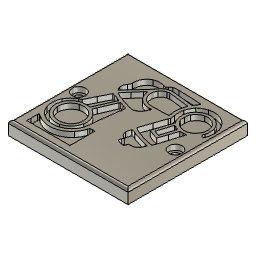
logo negative (Autodesk Fusion 360 design; units mm, degrees)
Autodesk Fusion 360 part; units mm, degrees
(part 1 of 2)
sketch "Sketch1" plane through (0, 0, 0) normal (0, 0, 1) x (1, 0, 0)
  line L0 (0, 0) -> (45, 0)
  line L1 (45, 0) -> (45, 45)
  line L2 (45, 45) -> (0, 45)
  line L3 (0, 45) -> (0, 0)
  dimension "d1" = 45
  dimension "d2" = 45
  constraint horizontal L0
  constraint vertical L1
  constraint horizontal L2
  constraint vertical L3
  constraint coincident L0.start L3.end
  measures "d1" distance of L0.start L0.end
  measures "d2" distance of L0.start L2.end
extrude "Extrude1" add sketch "Sketch1" along normal blind 5
sketch "Sketch2" plane through (0, 0, 5) normal (0, 0, 1) x (-1, 0, 0)
  line L0 (0, -45) -> (0, 0)
  line L1 (0, 0) -> (-45, 0)
  line L2 (-45, 0) -> (-45, -45)
  line L3 (-45, -45) -> (0, -45)
  spline S0 degree 3 poles (-20.168, -41.6441) (-19.9884, -41.5159) (-19.6164, -41.208) (-19.3214, -40.9258) knots 0 0 0 0 1 1 1 1
  line L4 (-19.3214, -40.9258) -> (-18.7954, -40.4255)
  line L5 (-18.7954, -40.4255) -> (-17.782, -40.6436)
  spline S1 degree 3 poles (-17.782, -40.6436) (-16.371, -40.9386) (-14.9471, -40.8488) (-13.985, -40.4127) knots 0 0 0 0 1 1 1 1
  spline S2 degree 3 poles (-13.985, -40.4127) (-12.2276, -39.6045) (-11.2014, -37.8086) (-11.1886, -35.5124) knots 0 0 0 0 1 1 1 1
  spline S3 degree 3 poles (-11.1886, -35.5124) (-11.1757, -34.9737) (-11.0988, -34.7299) (-10.6754, -34.1014) knots 0 0 0 0 1 1 1 1
  spline S4 degree 3 poles (-10.6754, -34.1014) (-10.1495, -33.3061) (-9.9443, -32.5236) (-10.0854, -31.8309) knots 0 0 0 0 1 1 1 1
  spline S5 degree 3 poles (-10.0854, -31.8309) (-10.1752, -31.3306) (-10.5472, -30.5609) (-10.6754, -30.5609) knots 0 0 0 0 1 1 1 1
  spline S6 degree 3 poles (-10.6754, -30.5609) (-10.7396, -30.5609) (-11.4964, -31.3178) (-12.3687, -32.2542) knots 0 0 0 0 1 1 1 1
  spline S7 degree 3 poles (-12.3687, -32.2542) (-13.241, -33.1778) (-14.5751, -34.6017) (-15.3319, -35.4098) knots 0 0 0 0 1 1 1 1
  spline S8 degree 3 poles (-15.3319, -35.4098) (-16.1016, -36.218) (-17.038, -37.2955) (-17.41, -37.8086) knots 0 0 0 0 1 1 1 1
  spline S9 degree 3 poles (-17.41, -37.8086) (-18.1797, -38.8477) (-19.052, -39.6558) (-19.7575, -40.0022) knots 0 0 0 0 1 1 1 1
  spline S10 degree 3 poles (-19.7575, -40.0022) (-20.5272, -40.3742) (-21.6689, -40.3614) (-25.1709, -39.938) knots 0 0 0 0 1 1 1 1
  spline S11 degree 3 poles (-25.1709, -39.938) (-26.9668, -39.72) (-28.737, -39.5019) (-29.0833, -39.4634) knots 0 0 0 0 1 1 1 1
  line L6 (-29.0833, -39.4634) -> (-29.7247, -39.3993)
  line L7 (-29.7247, -39.3993) -> (-30.3918, -40.3998)
  spline S12 degree 3 poles (-30.3918, -40.3998) (-30.969, -41.2593) (-31.0332, -41.4132) (-30.8408, -41.4774) knots 0 0 0 0 1 1 1 1
  spline S13 degree 3 poles (-30.8408, -41.4774) (-30.5329, -41.5928) (-24.7091, -41.8494) (-22.4001, -41.8494) knots 0 0 0 0 1 1 1 1
  spline S14 degree 3 poles (-22.4001, -41.8494) (-20.8351, -41.8494) (-20.4246, -41.8109) (-20.168, -41.6441) knots 0 0 0 0 1 1 1 1
  spline S15 degree 3 poles (-34.2786, -41.0412) (-33.1113, -40.6949) (-31.8798, -39.9637) (-31.2769, -39.271) knots 0 0 0 0 1 1 1 1
  spline S16 degree 3 poles (-31.2769, -39.271) (-30.6868, -38.5655) (-29.9685, -37.1801) (-29.7247, -36.2565) knots 0 0 0 0 1 1 1 1
  spline S17 degree 3 poles (-29.7247, -36.2565) (-29.5067, -35.4227) (-29.481, -33.7422) (-29.6734, -32.8699) knots 0 0 0 0 1 1 1 1
  spline S18 degree 3 poles (-29.6734, -32.8699) (-29.9172, -31.7539) (-29.9428, -31.3306) (-29.8145, -31.1766) knots 0 0 0 0 1 1 1 1
  spline S19 degree 3 poles (-29.8145, -31.1766) (-29.7504, -31.0869) (-29.6221, -30.8046) (-29.558, -30.5609) knots 0 0 0 0 1 1 1 1
  spline S20 degree 3 poles (-29.558, -30.5609) (-29.481, -30.3172) (-28.8396, -28.4058) (-28.1213, -26.3277) knots 0 0 0 0 1 1 1 1
  spline S21 degree 3 poles (-28.1213, -26.3277) (-26.7359, -22.3126) (-26.5434, -21.6969) (-26.6076, -21.6584) knots 0 0 0 0 1 1 1 1
  spline S22 degree 3 poles (-26.6076, -21.6584) (-27.3131, -21.1453) (-29.6991, -20.1576) (-31.4693, -19.6444) knots 0 0 0 0 1 1 1 1
  spline S23 degree 3 poles (-31.4693, -19.6444) (-32.9958, -19.2083) (-34.8559, -18.8363) (-35.0739, -18.9261) knots 0 0 0 0 1 1 1 1
  spline S24 degree 3 poles (-35.0739, -18.9261) (-35.2407, -18.9902) (-35.4973, -19.6829) (-36.3311, -22.4794) knots 0 0 0 0 1 1 1 1
  spline S25 degree 3 poles (-36.3311, -22.4794) (-36.5491, -23.2234) (-36.78, -23.9674) (-36.8442, -24.147) knots 0 0 0 0 1 1 1 1
  spline S26 degree 3 poles (-36.8442, -24.147) (-36.9083, -24.3266) (-37.1007, -24.9936) (-37.2931, -25.6222) knots 0 0 0 0 1 1 1 1
  spline S27 degree 3 poles (-37.2931, -25.6222) (-37.4856, -26.2636) (-37.7806, -27.2257) (-37.9602, -27.7901) knots 0 0 0 0 1 1 1 1
  spline S28 degree 3 poles (-37.9602, -27.7901) (-38.127, -28.3417) (-38.2424, -28.8163) (-38.2167, -28.8548) knots 0 0 0 0 1 1 1 1
  spline S29 degree 3 poles (-38.2167, -28.8548) (-38.1783, -28.8805) (-37.6395, -28.842) (-36.9981, -28.7522) knots 0 0 0 0 1 1 1 1
  line L8 (-36.9981, -28.7522) -> (-35.8436, -28.6111)
  line L9 (-35.8436, -28.6111) -> (-34.8045, -25.417)
  spline S30 degree 3 poles (-34.8045, -25.417) (-34.2273, -23.6724) (-33.7142, -22.21) (-33.6629, -22.1715) knots 0 0 0 0 1 1 1 1
  spline S31 degree 3 poles (-33.6629, -22.1715) (-33.5346, -22.0946) (-30.1865, -23.1849) (-30.0198, -23.3517) knots 0 0 0 0 1 1 1 1
  spline S32 degree 3 poles (-30.0198, -23.3517) (-29.93, -23.4415) (-30.3148, -24.7756) (-31.0588, -27.0076) knots 0 0 0 0 1 1 1 1
  line L10 (-31.0588, -27.0076) -> (-32.2262, -30.5353)
  line L11 (-32.2262, -30.5353) -> (-31.9055, -31.0869)
  spline S33 degree 3 poles (-31.9055, -31.0869) (-31.123, -32.4594) (-30.8536, -34.3964) (-31.2641, -35.769) knots 0 0 0 0 1 1 1 1
  spline S34 degree 3 poles (-31.2641, -35.769) (-31.713, -37.2827) (-33.3037, -38.7964) (-34.9457, -39.2966) knots 0 0 0 0 1 1 1 1
  spline S35 degree 3 poles (-34.9457, -39.2966) (-35.9077, -39.5917) (-37.306, -39.5917) (-38.2809, -39.2966) knots 0 0 0 0 1 1 1 1
  spline S36 degree 3 poles (-38.2809, -39.2966) (-39.5637, -38.899) (-40.9362, -37.5649) (-41.5007, -36.1667) knots 0 0 0 0 1 1 1 1
  spline S37 degree 3 poles (-41.5007, -36.1667) (-41.847, -35.32) (-41.8727, -33.3574) (-41.5391, -32.4979) knots 0 0 0 0 1 1 1 1
  spline S38 degree 3 poles (-41.5391, -32.4979) (-41.2185, -31.6384) (-41.2698, -31.4075) (-41.7829, -31.1638) knots 0 0 0 0 1 1 1 1
  spline S39 degree 3 poles (-41.7829, -31.1638) (-42.0394, -31.0484) (-42.2575, -30.9457) (-42.2832, -30.9457) knots 0 0 0 0 1 1 1 1
  spline S40 degree 3 poles (-42.2832, -30.9457) (-42.3088, -30.9457) (-42.5012, -31.3306) (-42.6937, -31.818) knots 0 0 0 0 1 1 1 1
  spline S41 degree 3 poles (-42.6937, -31.818) (-43.04, -32.6134) (-43.0657, -32.793) (-43.0528, -34.281) knots 0 0 0 0 1 1 1 1
  spline S42 degree 3 poles (-43.0528, -34.281) (-43.04, -35.6536) (-42.9887, -36.0127) (-42.7321, -36.7183) knots 0 0 0 0 1 1 1 1
  spline S43 degree 3 poles (-42.7321, -36.7183) (-41.4237, -40.2074) (-37.7806, -42.0675) (-34.2786, -41.0412) knots 0 0 0 0 1 1 1 1
  spline S44 degree 3 poles (-20.5657, -39.1299) (-19.8986, -38.9503) (-19.0648, -38.3217) (-18.6415, -37.6932) knots 0 0 0 0 1 1 1 1
  spline S45 degree 3 poles (-18.6415, -37.6932) (-17.2561, -35.6792) (-18.2439, -32.7545) (-20.6298, -31.8437) knots 0 0 0 0 1 1 1 1
  spline S46 degree 3 poles (-20.6298, -31.8437) (-21.3738, -31.5615) (-21.4636, -31.5615) (-24.9015, -31.6384) knots 0 0 0 0 1 1 1 1
  spline S47 degree 3 poles (-24.9015, -31.6384) (-26.8385, -31.6769) (-28.4804, -31.7667) (-28.5446, -31.8309) knots 0 0 0 0 1 1 1 1
  spline S48 degree 3 poles (-28.5446, -31.8309) (-28.6087, -31.895) (-28.5959, -32.344) (-28.4933, -32.9212) knots 0 0 0 0 1 1 1 1
  spline S49 degree 3 poles (-28.4933, -32.9212) (-28.288, -34.2553) (-28.4163, -35.8588) (-28.8396, -37.1929) knots 0 0 0 0 1 1 1 1
  spline S50 degree 3 poles (-28.8396, -37.1929) (-29.032, -37.783) (-29.1603, -38.2833) (-29.1347, -38.3089) knots 0 0 0 0 1 1 1 1
  spline S51 degree 3 poles (-29.1347, -38.3089) (-29.0449, -38.3987) (-21.9254, -39.2838) (-21.4508, -39.271) knots 0 0 0 0 1 1 1 1
  spline S52 degree 3 poles (-21.4508, -39.271) (-21.2071, -39.271) (-20.8094, -39.2069) (-20.5657, -39.1299) knots 0 0 0 0 1 1 1 1
  spline S53 degree 3 poles (-35.4844, -38.3987) (-34.253, -38.1037) (-33.1241, -37.2057) (-32.5084, -36.0127) knots 0 0 0 0 1 1 1 1
  spline S54 degree 3 poles (-32.5084, -36.0127) (-32.2005, -35.4483) (-32.162, -35.2302) (-32.162, -34.0886) knots 0 0 0 0 1 1 1 1
  spline S55 degree 3 poles (-32.162, -34.0886) (-32.162, -32.9341) (-32.2005, -32.7416) (-32.5212, -32.1259) knots 0 0 0 0 1 1 1 1
  spline S56 degree 3 poles (-32.5212, -32.1259) (-33.65, -29.9837) (-36.1643, -29.137) (-38.3194, -30.1761) knots 0 0 0 0 1 1 1 1
  spline S57 degree 3 poles (-38.3194, -30.1761) (-39.0762, -30.5481) (-39.9742, -31.4717) (-40.3975, -32.3311) knots 0 0 0 0 1 1 1 1
  spline S58 degree 3 poles (-40.3975, -32.3311) (-40.7053, -32.9725) (-40.7567, -33.2163) (-40.7567, -34.2168) knots 0 0 0 0 1 1 1 1
  spline S59 degree 3 poles (-40.7567, -34.2168) (-40.7567, -35.2431) (-40.7182, -35.4611) (-40.3718, -36.1154) knots 0 0 0 0 1 1 1 1
  spline S60 degree 3 poles (-40.3718, -36.1154) (-39.4739, -37.8984) (-37.4086, -38.8477) (-35.4844, -38.3987) knots 0 0 0 0 1 1 1 1
  spline S61 degree 3 poles (-16.0631, -34.7428) (-15.6783, -34.2938) (-14.7034, -33.1778) (-13.8952, -32.2798) knots 0 0 0 0 1 1 1 1
  spline S62 degree 3 poles (-13.8952, -32.2798) (-11.9967, -30.1248) (-11.6632, -29.6758) (-11.8428, -29.4577) knots 0 0 0 0 1 1 1 1
  spline S63 degree 3 poles (-11.8428, -29.4577) (-12.0224, -29.2396) (-14.0363, -28.4572) (-16.5762, -27.6105) knots 0 0 0 0 1 1 1 1
  spline S64 degree 3 poles (-16.5762, -27.6105) (-19.0007, -26.8024) (-20.0141, -26.6741) (-20.8351, -27.0846) knots 0 0 0 0 1 1 1 1
  spline S65 degree 3 poles (-20.8351, -27.0846) (-21.9639, -27.6233) (-22.9517, -28.9061) (-23.1697, -30.0991) knots 0 0 0 0 1 1 1 1
  line L12 (-23.1697, -30.0991) -> (-23.2595, -30.5994)
  line L13 (-23.2595, -30.5994) -> (-22.5283, -30.5224)
  spline S66 degree 3 poles (-22.5283, -30.5224) (-21.0531, -30.3685) (-19.6036, -30.8944) (-18.4876, -31.9848) knots 0 0 0 0 1 1 1 1
  spline S67 degree 3 poles (-18.4876, -31.9848) (-17.7564, -32.7032) (-17.115, -33.9603) (-16.9996, -34.9352) knots 0 0 0 0 1 1 1 1
  spline S68 degree 3 poles (-16.9996, -34.9352) (-16.9611, -35.2815) (-16.8841, -35.5638) (-16.8456, -35.5509) knots 0 0 0 0 1 1 1 1
  spline S69 degree 3 poles (-16.8456, -35.5509) (-16.8071, -35.5509) (-16.448, -35.1789) (-16.0631, -34.7428) knots 0 0 0 0 1 1 1 1
  spline S70 degree 3 poles (-32.9573, -29.5732) (-32.7649, -29.2525) (-31.1871, -24.224) (-31.2256, -24.0572) knots 0 0 0 0 1 1 1 1
  spline S71 degree 3 poles (-31.2256, -24.0572) (-31.2641, -23.852) (-32.9317, -23.2747) (-33.0728, -23.4158) knots 0 0 0 0 1 1 1 1
  spline S72 degree 3 poles (-33.0728, -23.4158) (-33.1498, -23.4928) (-34.5352, -27.8414) (-34.7148, -28.5469) knots 0 0 0 0 1 1 1 1
  spline S73 degree 3 poles (-34.7148, -28.5469) (-34.7789, -28.842) (-34.7532, -28.919) (-34.471, -29.0216) knots 0 0 0 0 1 1 1 1
  spline S74 degree 3 poles (-34.471, -29.0216) (-34.3043, -29.0857) (-33.9066, -29.2653) (-33.6116, -29.4064) knots 0 0 0 0 1 1 1 1
  spline S75 degree 3 poles (-33.6116, -29.4064) (-32.9958, -29.7014) (-33.0343, -29.6886) (-32.9573, -29.5732) knots 0 0 0 0 1 1 1 1
  spline S76 degree 3 poles (-10.9577, -28.3417) (-10.8807, -28.2519) (-9.9827, -26.4945) (-8.9565, -24.442) knots 0 0 0 0 1 1 1 1
  line L14 (-8.9565, -24.442) -> (-7.0837, -20.6835)
  line L15 (-7.0837, -20.6835) -> (-6.2114, -20.273)
  spline S77 degree 3 poles (-6.2114, -20.273) (-5.0056, -19.6829) (-3.6971, -18.3617) (-3.0686, -17.0917) knots 0 0 0 0 1 1 1 1
  spline S78 degree 3 poles (-3.0686, -17.0917) (-2.2476, -15.4241) (-2.145, -13.5256) (-2.7863, -11.6784) knots 0 0 0 0 1 1 1 1
  spline S79 degree 3 poles (-2.7863, -11.6784) (-3.4534, -9.767) (-5.0953, -8.1892) (-7.1606, -7.458) knots 0 0 0 0 1 1 1 1
  spline S80 degree 3 poles (-7.1606, -7.458) (-8.1355, -7.1245) (-10.1238, -6.9962) (-11.0731, -7.2143) knots 0 0 0 0 1 1 1 1
  spline S81 degree 3 poles (-11.0731, -7.2143) (-12.3815, -7.5093) (-13.613, -8.202) (-14.6008, -9.1898) knots 0 0 0 0 1 1 1 1
  spline S82 degree 3 poles (-14.6008, -9.1898) (-16.0503, -10.6393) (-16.5762, -11.9349) (-16.7687, -14.5903) knots 0 0 0 0 1 1 1 1
  spline S83 degree 3 poles (-16.7687, -14.5903) (-16.8328, -15.578) (-17.115, -17.9383) (-17.41, -20.0421) knots 0 0 0 0 1 1 1 1
  spline S84 degree 3 poles (-17.41, -20.0421) (-17.4485, -20.3628) (-17.564, -21.1966) (-17.6538, -21.9021) knots 0 0 0 0 1 1 1 1
  spline S85 degree 3 poles (-17.6538, -21.9021) (-17.7564, -22.6077) (-17.9103, -23.7365) (-18.0001, -24.4164) knots 0 0 0 0 1 1 1 1
  spline S86 degree 3 poles (-18.0001, -24.4164) (-18.0899, -25.0834) (-18.1284, -25.7248) (-18.0899, -25.8403) knots 0 0 0 0 1 1 1 1
  spline S87 degree 3 poles (-18.0899, -25.8403) (-18.0386, -25.9557) (-17.4357, -26.2251) (-16.6404, -26.4945) knots 0 0 0 0 1 1 1 1
  line L16 (-16.6404, -26.4945) -> (-15.2806, -26.9563)
  line L17 (-15.2806, -26.9563) -> (-15.101, -26.5458)
  spline S88 degree 3 poles (-15.101, -26.5458) (-14.8188, -25.9172) (-13.2923, -22.3383) (-12.6381, -20.7476) knots 0 0 0 0 1 1 1 1
  line L18 (-12.6381, -20.7476) -> (-12.048, -19.3494)
  line L19 (-12.048, -19.3494) -> (-12.3559, -19.1442)
  spline S89 degree 3 poles (-12.3559, -19.1442) (-14.7419, -17.5792) (-15.7296, -15.5267) (-15.3063, -13.051) knots 0 0 0 0 1 1 1 1
  spline S90 degree 3 poles (-15.3063, -13.051) (-14.9086, -10.7676) (-13.0742, -8.8691) (-10.8294, -8.3816) knots 0 0 0 0 1 1 1 1
  spline S91 degree 3 poles (-10.8294, -8.3816) (-7.4685, -7.6761) (-4.1333, -9.9338) (-3.6202, -13.2819) knots 0 0 0 0 1 1 1 1
  spline S92 degree 3 poles (-3.6202, -13.2819) (-3.1968, -16.0527) (-4.9542, -18.7722) (-7.725, -19.5803) knots 0 0 0 0 1 1 1 1
  spline S93 degree 3 poles (-7.725, -19.5803) (-8.2125, -19.7342) (-8.8282, -19.7856) (-9.7134, -19.7727) knots 0 0 0 0 1 1 1 1
  line L20 (-9.7134, -19.7727) -> (-10.9961, -19.7342)
  line L21 (-10.9961, -19.7342) -> (-11.4066, -20.5681)
  spline S94 degree 3 poles (-11.4066, -20.5681) (-11.8941, -21.543) (-14.2672, -27.0333) (-14.2672, -27.2) knots 0 0 0 0 1 1 1 1
  spline S95 degree 3 poles (-14.2672, -27.2) (-14.2672, -27.2513) (-13.8439, -27.4566) (-13.3436, -27.6362) knots 0 0 0 0 1 1 1 1
  spline S96 degree 3 poles (-13.3436, -27.6362) (-12.8305, -27.8158) (-12.1122, -28.0851) (-11.7402, -28.2263) knots 0 0 0 0 1 1 1 1
  spline S97 degree 3 poles (-11.7402, -28.2263) (-11.2399, -28.4315) (-11.0475, -28.4572) (-10.9577, -28.3417) knots 0 0 0 0 1 1 1 1
  spline S98 degree 3 poles (-26.2612, -20.1447) (-26.0175, -19.4905) (-25.8123, -18.6311) (-25.8123, -18.2719) knots 0 0 0 0 1 1 1 1
  spline S99 degree 3 poles (-25.8123, -18.2719) (-25.8123, -17.5663) (-26.3767, -16.6171) (-27.0052, -16.3092) knots 0 0 0 0 1 1 1 1
  spline S100 degree 3 poles (-27.0052, -16.3092) (-27.3003, -16.1553) (-27.5568, -16.0142) (-27.5825, -16.0014) knots 0 0 0 0 1 1 1 1
  spline S101 degree 3 poles (-27.5825, -16.0014) (-27.5953, -15.9885) (-27.5055, -15.6678) (-27.3516, -15.3086) knots 0 0 0 0 1 1 1 1
  spline S102 degree 3 poles (-27.3516, -15.3086) (-26.9283, -14.2311) (-26.9539, -14.2055) (-28.1597, -13.8335) knots 0 0 0 0 1 1 1 1
  spline S103 degree 3 poles (-28.1597, -13.8335) (-29.8274, -13.3203) (-29.8017, -13.3203) (-30.1352, -14.1413) knots 0 0 0 0 1 1 1 1
  line L22 (-30.1352, -14.1413) -> (-30.4174, -14.8468)
  line L23 (-30.4174, -14.8468) -> (-31.123, -14.8084)
  spline S104 degree 3 poles (-31.123, -14.8084) (-32.0722, -14.7571) (-32.8162, -15.0906) (-33.4448, -15.8474) knots 0 0 0 0 1 1 1 1
  spline S105 degree 3 poles (-33.4448, -15.8474) (-33.8553, -16.3349) (-34.4069, -17.4252) (-34.4069, -17.7459) knots 0 0 0 0 1 1 1 1
  spline S106 degree 3 poles (-34.4069, -17.7459) (-34.4069, -17.7972) (-34.0221, -17.8999) (-33.5474, -17.9897) knots 0 0 0 0 1 1 1 1
  spline S107 degree 3 poles (-33.5474, -17.9897) (-32.4314, -18.1821) (-29.2758, -19.157) (-27.7236, -19.7984) knots 0 0 0 0 1 1 1 1
  spline S108 degree 3 poles (-27.7236, -19.7984) (-26.351, -20.3628) (-26.3382, -20.3628) (-26.2612, -20.1447) knots 0 0 0 0 1 1 1 1
  spline S109 degree 3 poles (-8.1099, -18.5669) (-5.9805, -17.9768) (-4.4668, -15.7705) (-4.7105, -13.6026) knots 0 0 0 0 1 1 1 1
  spline S110 degree 3 poles (-4.7105, -13.6026) (-4.826, -12.5892) (-5.5187, -11.2166) (-6.2242, -10.6008) knots 0 0 0 0 1 1 1 1
  spline S111 degree 3 poles (-6.2242, -10.6008) (-7.6609, -9.3437) (-9.8929, -8.9974) (-11.599, -9.7542) knots 0 0 0 0 1 1 1 1
  spline S112 degree 3 poles (-11.599, -9.7542) (-14.4981, -11.0242) (-15.178, -15.0393) (-12.8947, -17.3226) knots 0 0 0 0 1 1 1 1
  spline S113 degree 3 poles (-12.8947, -17.3226) (-11.6504, -18.5669) (-9.8288, -19.0415) (-8.1099, -18.5669) knots 0 0 0 0 1 1 1 1
  spline S114 degree 3 poles (-17.9488, -12.6405) (-17.9103, -12.5763) (-17.8462, -12.3326) (-17.7949, -12.0889) knots 0 0 0 0 1 1 1 1
  spline S115 degree 3 poles (-17.7949, -12.0889) (-17.6281, -11.2679) (-16.7302, -9.5874) (-16.0375, -8.805) knots 0 0 0 0 1 1 1 1
  spline S116 degree 3 poles (-16.0375, -8.805) (-13.0358, -5.3928) (-8.2382, -4.8412) (-4.3898, -7.458) knots 0 0 0 0 1 1 1 1
  line L24 (-4.3898, -7.458) -> (-3.6586, -7.9583)
  line L25 (-3.6586, -7.9583) -> (-3.5688, -7.3041)
  spline S117 degree 3 poles (-3.5688, -7.3041) (-3.5304, -6.9321) (-3.4919, -5.9059) (-3.4919, -5.0079) knots 0 0 0 0 1 1 1 1
  line L26 (-3.4919, -5.0079) -> (-3.4919, -3.366)
  line L27 (-3.4919, -3.366) -> (-11.6375, -3.366)
  line L28 (-11.6375, -3.366) -> (-19.7832, -3.366)
  line L29 (-19.7832, -3.366) -> (-19.7832, -8.0481)
  line L30 (-19.7832, -8.0481) -> (-19.7832, -12.7303)
  line L31 (-19.7832, -12.7303) -> (-18.8981, -12.7303)
  spline S118 degree 3 poles (-18.8981, -12.7303) (-18.3978, -12.7303) (-17.9745, -12.6918) (-17.9488, -12.6405) knots 0 0 0 0 1 1 1 1
  measures "d7" diameter of S13.end
  measures "d11" diameter of S13.end
extrude "Extrude2" cut sketch "Sketch2" against normal blind 2 contours S0 L4 L5 S1 S2 S3 S4 S5 S6 S7 S8 S9 S10 S11 L6 L7 S12 S13 S14 | S15 S16 S17 S18 S19 S20 S21 S22 S23 S24 S25 S26 S27 S28 S29 L8 L9 S30 S31 S32 L10 L11 S33 S34 S35 S36 S37 S38 S39 S40 S41 S42 S43 | S44 S45 S46 S47 S48 S49 S50 S51 S52 | S53 S54 S55 S56 S57 S58 S59 S60 | S61 S62 S63 S64 S65 L12 L13 S66 S67 S68 S69 | S70 S71 S72 S73 S74 S75 | S76 L14 L15 S77 S78 S79 S80 S81 S82 S83 S84 S85 S86 S87 L16 L17 S88 L18 L19 S89 S90 S91 S92 S93 L20 L21 S94 S95 S96 S97 | S98 S99 S100 S101 S102 S103 L22 L23 S104 S105 S106 S107 S108 | S109 S110 S111 S112 S113 | S114 S115 S116 L24 L25 S117 L26 L27 L28 L29 L30 L31 S118
sketch "Sketch3" plane through (0, 0, 5) normal (0, 0, 1) x (-1, 0, 0)
  spline S0 degree 3 poles (-31.2769, -39.271) (-31.8798, -39.9637) (-33.1113, -40.6949) (-34.2786, -41.0412) knots -1 -1 -1 -1 0 0 0 0
  spline S1 degree 3 poles (-34.2786, -41.0412) (-37.7806, -42.0675) (-41.4237, -40.2074) (-42.7321, -36.7183) knots -1 -1 -1 -1 0 0 0 0
  spline S2 degree 3 poles (-42.7321, -36.7183) (-42.9887, -36.0127) (-43.04, -35.6536) (-43.0528, -34.281) knots -1 -1 -1 -1 0 0 0 0
  spline S3 degree 3 poles (-43.0528, -34.281) (-43.0657, -32.793) (-43.04, -32.6134) (-42.6937, -31.818) knots -1 -1 -1 -1 0 0 0 0
  spline S4 degree 3 poles (-42.6937, -31.818) (-42.5012, -31.3306) (-42.3088, -30.9457) (-42.2832, -30.9457) knots -1 -1 -1 -1 0 0 0 0
  spline S5 degree 3 poles (-42.2832, -30.9457) (-42.2575, -30.9457) (-42.0394, -31.0484) (-41.7829, -31.1638) knots -1 -1 -1 -1 0 0 0 0
  spline S6 degree 3 poles (-41.7829, -31.1638) (-41.2698, -31.4075) (-41.2185, -31.6384) (-41.5391, -32.4979) knots -1 -1 -1 -1 0 0 0 0
  spline S7 degree 3 poles (-41.5391, -32.4979) (-41.8727, -33.3574) (-41.847, -35.32) (-41.5007, -36.1667) knots -1 -1 -1 -1 0 0 0 0
  spline S8 degree 3 poles (-41.5007, -36.1667) (-40.9362, -37.5649) (-39.5637, -38.899) (-38.2809, -39.2966) knots -1 -1 -1 -1 0 0 0 0
  spline S9 degree 3 poles (-38.2809, -39.2966) (-37.306, -39.5917) (-35.9077, -39.5917) (-34.9457, -39.2966) knots -1 -1 -1 -1 0 0 0 0
  spline S10 degree 3 poles (-34.9457, -39.2966) (-33.3037, -38.7964) (-31.713, -37.2827) (-31.2641, -35.769) knots -1 -1 -1 -1 0 0 0 0
  spline S11 degree 3 poles (-31.2641, -35.769) (-30.8536, -34.3964) (-31.123, -32.4594) (-31.9055, -31.0869) knots -1 -1 -1 -1 0 0 0 0
  line L0 (-31.9055, -31.0869) -> (-32.2262, -30.5353)
  line L1 (-32.2262, -30.5353) -> (-31.0588, -27.0076)
  spline S12 degree 3 poles (-31.0588, -27.0076) (-30.3148, -24.7756) (-29.93, -23.4415) (-30.0198, -23.3517) knots -1 -1 -1 -1 0 0 0 0
  spline S13 degree 3 poles (-30.0198, -23.3517) (-30.1865, -23.1849) (-33.5346, -22.0946) (-33.6629, -22.1715) knots -1 -1 -1 -1 0 0 0 0
  spline S14 degree 3 poles (-33.6629, -22.1715) (-33.7142, -22.21) (-34.2273, -23.6724) (-34.8045, -25.417) knots -1 -1 -1 -1 0 0 0 0
  line L2 (-34.8045, -25.417) -> (-35.8436, -28.6111)
  line L3 (-35.8436, -28.6111) -> (-36.9981, -28.7522)
  spline S15 degree 3 poles (-36.9981, -28.7522) (-37.6395, -28.842) (-38.1783, -28.8805) (-38.2167, -28.8548) knots -1 -1 -1 -1 0 0 0 0
  spline S16 degree 3 poles (-38.2167, -28.8548) (-38.2424, -28.8163) (-38.127, -28.3417) (-37.9602, -27.7901) knots -1 -1 -1 -1 0 0 0 0
  spline S17 degree 3 poles (-37.9602, -27.7901) (-37.7806, -27.2257) (-37.4856, -26.2636) (-37.2931, -25.6222) knots -1 -1 -1 -1 0 0 0 0
  spline S18 degree 3 poles (-37.2931, -25.6222) (-37.1007, -24.9936) (-36.9083, -24.3266) (-36.8442, -24.147) knots -1 -1 -1 -1 0 0 0 0
  spline S19 degree 3 poles (-36.8442, -24.147) (-36.78, -23.9674) (-36.5491, -23.2234) (-36.3311, -22.4794) knots -1 -1 -1 -1 0 0 0 0
  spline S20 degree 3 poles (-36.3311, -22.4794) (-35.4973, -19.6829) (-35.2407, -18.9902) (-35.0739, -18.9261) knots -1 -1 -1 -1 0 0 0 0
  spline S21 degree 3 poles (-35.0739, -18.9261) (-34.8559, -18.8363) (-32.9958, -19.2083) (-31.4693, -19.6444) knots -1 -1 -1 -1 0 0 0 0
  spline S22 degree 3 poles (-31.4693, -19.6444) (-29.6991, -20.1576) (-27.3131, -21.1453) (-26.6076, -21.6584) knots -1 -1 -1 -1 0 0 0 0
  spline S23 degree 3 poles (-26.6076, -21.6584) (-26.5434, -21.6969) (-26.7359, -22.3126) (-28.1213, -26.3277) knots -1 -1 -1 -1 0 0 0 0
  spline S24 degree 3 poles (-28.1213, -26.3277) (-28.8396, -28.4058) (-29.481, -30.3172) (-29.558, -30.5609) knots -1 -1 -1 -1 0 0 0 0
  spline S25 degree 3 poles (-29.558, -30.5609) (-29.6221, -30.8046) (-29.7504, -31.0869) (-29.8145, -31.1766) knots -1 -1 -1 -1 0 0 0 0
  spline S26 degree 3 poles (-29.8145, -31.1766) (-29.9428, -31.3306) (-29.9172, -31.7539) (-29.6734, -32.8699) knots -1 -1 -1 -1 0 0 0 0
  spline S27 degree 3 poles (-29.6734, -32.8699) (-29.481, -33.7422) (-29.5067, -35.4227) (-29.7247, -36.2565) knots -1 -1 -1 -1 0 0 0 0
  spline S28 degree 3 poles (-29.7247, -36.2565) (-29.9685, -37.1801) (-30.6868, -38.5655) (-31.2769, -39.271) knots -1 -1 -1 -1 0 0 0 0
  spline S29 degree 3 poles (-13.8952, -32.2798) (-14.7034, -33.1778) (-15.6783, -34.2938) (-16.0631, -34.7428) knots -1 -1 -1 -1 0 0 0 0
  spline S30 degree 3 poles (-16.0631, -34.7428) (-16.448, -35.1789) (-16.8071, -35.5509) (-16.8456, -35.5509) knots -1 -1 -1 -1 0 0 0 0
  spline S31 degree 3 poles (-16.8456, -35.5509) (-16.8841, -35.5638) (-16.9611, -35.2815) (-16.9996, -34.9352) knots -1 -1 -1 -1 0 0 0 0
  spline S32 degree 3 poles (-16.9996, -34.9352) (-17.115, -33.9603) (-17.7564, -32.7032) (-18.4876, -31.9848) knots -1 -1 -1 -1 0 0 0 0
  spline S33 degree 3 poles (-18.4876, -31.9848) (-19.6036, -30.8944) (-21.0531, -30.3685) (-22.5283, -30.5224) knots -1 -1 -1 -1 0 0 0 0
  line L4 (-22.5283, -30.5224) -> (-23.2595, -30.5994)
  line L5 (-23.2595, -30.5994) -> (-23.1697, -30.0991)
  spline S34 degree 3 poles (-23.1697, -30.0991) (-22.9517, -28.9061) (-21.9639, -27.6233) (-20.8351, -27.0846) knots -1 -1 -1 -1 0 0 0 0
  spline S35 degree 3 poles (-20.8351, -27.0846) (-20.0141, -26.6741) (-19.0007, -26.8024) (-16.5762, -27.6105) knots -1 -1 -1 -1 0 0 0 0
  spline S36 degree 3 poles (-16.5762, -27.6105) (-14.0363, -28.4572) (-12.0224, -29.2396) (-11.8428, -29.4577) knots -1 -1 -1 -1 0 0 0 0
  spline S37 degree 3 poles (-11.8428, -29.4577) (-11.6632, -29.6758) (-11.9967, -30.1248) (-13.8952, -32.2798) knots -1 -1 -1 -1 0 0 0 0
  spline S38 degree 3 poles (-8.9565, -24.442) (-9.9827, -26.4945) (-10.8807, -28.2519) (-10.9577, -28.3417) knots -1 -1 -1 -1 0 0 0 0
  spline S39 degree 3 poles (-10.9577, -28.3417) (-11.0475, -28.4572) (-11.2399, -28.4315) (-11.7402, -28.2263) knots -1 -1 -1 -1 0 0 0 0
  spline S40 degree 3 poles (-11.7402, -28.2263) (-12.1122, -28.0851) (-12.8305, -27.8158) (-13.3436, -27.6362) knots -1 -1 -1 -1 0 0 0 0
  spline S41 degree 3 poles (-13.3436, -27.6362) (-13.8439, -27.4566) (-14.2672, -27.2513) (-14.2672, -27.2) knots -1 -1 -1 -1 0 0 0 0
  spline S42 degree 3 poles (-14.2672, -27.2) (-14.2672, -27.0333) (-11.8941, -21.543) (-11.4066, -20.5681) knots -1 -1 -1 -1 0 0 0 0
  line L6 (-11.4066, -20.5681) -> (-10.9961, -19.7342)
  line L7 (-10.9961, -19.7342) -> (-9.7134, -19.7727)
  spline S43 degree 3 poles (-9.7134, -19.7727) (-8.8282, -19.7856) (-8.2125, -19.7342) (-7.725, -19.5803) knots -1 -1 -1 -1 0 0 0 0
  spline S44 degree 3 poles (-7.725, -19.5803) (-4.9542, -18.7722) (-3.1968, -16.0527) (-3.6202, -13.2819) knots -1 -1 -1 -1 0 0 0 0
  spline S45 degree 3 poles (-3.6202, -13.2819) (-4.1333, -9.9338) (-7.4685, -7.6761) (-10.8294, -8.3816) knots -1 -1 -1 -1 0 0 0 0
  spline S46 degree 3 poles (-10.8294, -8.3816) (-13.0742, -8.8691) (-14.9086, -10.7676) (-15.3063, -13.051) knots -1 -1 -1 -1 0 0 0 0
  spline S47 degree 3 poles (-15.3063, -13.051) (-15.7296, -15.5267) (-14.7419, -17.5792) (-12.3559, -19.1442) knots -1 -1 -1 -1 0 0 0 0
  line L8 (-12.3559, -19.1442) -> (-12.048, -19.3494)
  line L9 (-12.048, -19.3494) -> (-12.6381, -20.7476)
  spline S48 degree 3 poles (-12.6381, -20.7476) (-13.2923, -22.3383) (-14.8188, -25.9172) (-15.101, -26.5458) knots -1 -1 -1 -1 0 0 0 0
  line L10 (-15.101, -26.5458) -> (-15.2806, -26.9563)
  line L11 (-15.2806, -26.9563) -> (-16.6404, -26.4945)
  spline S49 degree 3 poles (-16.6404, -26.4945) (-17.4357, -26.2251) (-18.0386, -25.9557) (-18.0899, -25.8403) knots -1 -1 -1 -1 0 0 0 0
  spline S50 degree 3 poles (-18.0899, -25.8403) (-18.1284, -25.7248) (-18.0899, -25.0834) (-18.0001, -24.4164) knots -1 -1 -1 -1 0 0 0 0
  spline S51 degree 3 poles (-18.0001, -24.4164) (-17.9103, -23.7365) (-17.7564, -22.6077) (-17.6538, -21.9021) knots -1 -1 -1 -1 0 0 0 0
  spline S52 degree 3 poles (-17.6538, -21.9021) (-17.564, -21.1966) (-17.4485, -20.3628) (-17.41, -20.0421) knots -1 -1 -1 -1 0 0 0 0
  spline S53 degree 3 poles (-17.41, -20.0421) (-17.115, -17.9383) (-16.8328, -15.578) (-16.7687, -14.5903) knots -1 -1 -1 -1 0 0 0 0
  spline S54 degree 3 poles (-16.7687, -14.5903) (-16.5762, -11.9349) (-16.0503, -10.6393) (-14.6008, -9.1898) knots -1 -1 -1 -1 0 0 0 0
  spline S55 degree 3 poles (-14.6008, -9.1898) (-13.613, -8.202) (-12.3815, -7.5093) (-11.0731, -7.2143) knots -1 -1 -1 -1 0 0 0 0
  spline S56 degree 3 poles (-11.0731, -7.2143) (-10.1238, -6.9962) (-8.1355, -7.1245) (-7.1606, -7.458) knots -1 -1 -1 -1 0 0 0 0
  spline S57 degree 3 poles (-7.1606, -7.458) (-5.0953, -8.1892) (-3.4534, -9.767) (-2.7863, -11.6784) knots -1 -1 -1 -1 0 0 0 0
  spline S58 degree 3 poles (-2.7863, -11.6784) (-2.145, -13.5256) (-2.2476, -15.4241) (-3.0686, -17.0917) knots -1 -1 -1 -1 0 0 0 0
  spline S59 degree 3 poles (-3.0686, -17.0917) (-3.6971, -18.3617) (-5.0056, -19.6829) (-6.2114, -20.273) knots -1 -1 -1 -1 0 0 0 0
  line L12 (-6.2114, -20.273) -> (-7.0837, -20.6835)
  line L13 (-7.0837, -20.6835) -> (-8.9565, -24.442)
  spline S60 degree 3 poles (-19.3214, -40.9258) (-19.6164, -41.208) (-19.9884, -41.5159) (-20.168, -41.6441) knots -1 -1 -1 -1 0 0 0 0
  spline S61 degree 3 poles (-20.168, -41.6441) (-20.4246, -41.8109) (-20.8351, -41.8494) (-22.4001, -41.8494) knots -1 -1 -1 -1 0 0 0 0
  spline S62 degree 3 poles (-22.4001, -41.8494) (-24.7091, -41.8494) (-30.5329, -41.5928) (-30.8408, -41.4774) knots -1 -1 -1 -1 0 0 0 0
  spline S63 degree 3 poles (-30.8408, -41.4774) (-31.0332, -41.4132) (-30.969, -41.2593) (-30.3918, -40.3998) knots -1 -1 -1 -1 0 0 0 0
  line L14 (-30.3918, -40.3998) -> (-29.7247, -39.3993)
  line L15 (-29.7247, -39.3993) -> (-29.0833, -39.4634)
  spline S64 degree 3 poles (-29.0833, -39.4634) (-28.737, -39.5019) (-26.9668, -39.72) (-25.1709, -39.938) knots -1 -1 -1 -1 0 0 0 0
  spline S65 degree 3 poles (-25.1709, -39.938) (-21.6689, -40.3614) (-20.5272, -40.3742) (-19.7575, -40.0022) knots -1 -1 -1 -1 0 0 0 0
  spline S66 degree 3 poles (-19.7575, -40.0022) (-19.052, -39.6558) (-18.1797, -38.8477) (-17.41, -37.8086) knots -1 -1 -1 -1 0 0 0 0
  spline S67 degree 3 poles (-17.41, -37.8086) (-17.038, -37.2955) (-16.1016, -36.218) (-15.3319, -35.4098) knots -1 -1 -1 -1 0 0 0 0
  spline S68 degree 3 poles (-15.3319, -35.4098) (-14.5751, -34.6017) (-13.241, -33.1778) (-12.3687, -32.2542) knots -1 -1 -1 -1 0 0 0 0
  spline S69 degree 3 poles (-12.3687, -32.2542) (-11.4964, -31.3178) (-10.7396, -30.5609) (-10.6754, -30.5609) knots -1 -1 -1 -1 0 0 0 0
  spline S70 degree 3 poles (-10.6754, -30.5609) (-10.5472, -30.5609) (-10.1752, -31.3306) (-10.0854, -31.8309) knots -1 -1 -1 -1 0 0 0 0
  spline S71 degree 3 poles (-10.0854, -31.8309) (-9.9443, -32.5236) (-10.1495, -33.3061) (-10.6754, -34.1014) knots -1 -1 -1 -1 0 0 0 0
  spline S72 degree 3 poles (-10.6754, -34.1014) (-11.0988, -34.7299) (-11.1757, -34.9737) (-11.1886, -35.5124) knots -1 -1 -1 -1 0 0 0 0
  spline S73 degree 3 poles (-11.1886, -35.5124) (-11.2014, -37.8086) (-12.2276, -39.6045) (-13.985, -40.4127) knots -1 -1 -1 -1 0 0 0 0
  spline S74 degree 3 poles (-13.985, -40.4127) (-14.9471, -40.8488) (-16.371, -40.9386) (-17.782, -40.6436) knots -1 -1 -1 -1 0 0 0 0
  line L16 (-17.782, -40.6436) -> (-18.7954, -40.4255)
  line L17 (-18.7954, -40.4255) -> (-19.3214, -40.9258)
  spline S75 degree 3 poles (-31.2256, -24.0572) (-31.1871, -24.224) (-32.7649, -29.2525) (-32.9573, -29.5732) knots -1 -1 -1 -1 0 0 0 0
  spline S76 degree 3 poles (-32.9573, -29.5732) (-33.0343, -29.6886) (-32.9958, -29.7014) (-33.6116, -29.4064) knots -1 -1 -1 -1 0 0 0 0
  spline S77 degree 3 poles (-33.6116, -29.4064) (-33.9066, -29.2653) (-34.3043, -29.0857) (-34.471, -29.0216) knots -1 -1 -1 -1 0 0 0 0
  spline S78 degree 3 poles (-34.471, -29.0216) (-34.7532, -28.919) (-34.7789, -28.842) (-34.7148, -28.5469) knots -1 -1 -1 -1 0 0 0 0
  spline S79 degree 3 poles (-34.7148, -28.5469) (-34.5352, -27.8414) (-33.1498, -23.4928) (-33.0728, -23.4158) knots -1 -1 -1 -1 0 0 0 0
  spline S80 degree 3 poles (-33.0728, -23.4158) (-32.9317, -23.2747) (-31.2641, -23.852) (-31.2256, -24.0572) knots -1 -1 -1 -1 0 0 0 0
  spline S81 degree 3 poles (-32.5084, -36.0127) (-33.1241, -37.2057) (-34.253, -38.1037) (-35.4844, -38.3987) knots -1 -1 -1 -1 0 0 0 0
  spline S82 degree 3 poles (-35.4844, -38.3987) (-37.4086, -38.8477) (-39.4739, -37.8984) (-40.3718, -36.1154) knots -1 -1 -1 -1 0 0 0 0
  spline S83 degree 3 poles (-40.3718, -36.1154) (-40.7182, -35.4611) (-40.7567, -35.2431) (-40.7567, -34.2168) knots -1 -1 -1 -1 0 0 0 0
  spline S84 degree 3 poles (-40.7567, -34.2168) (-40.7567, -33.2163) (-40.7053, -32.9725) (-40.3975, -32.3311) knots -1 -1 -1 -1 0 0 0 0
  spline S85 degree 3 poles (-40.3975, -32.3311) (-39.9742, -31.4717) (-39.0762, -30.5481) (-38.3194, -30.1761) knots -1 -1 -1 -1 0 0 0 0
  spline S86 degree 3 poles (-38.3194, -30.1761) (-36.1643, -29.137) (-33.65, -29.9837) (-32.5212, -32.1259) knots -1 -1 -1 -1 0 0 0 0
  spline S87 degree 3 poles (-32.5212, -32.1259) (-32.2005, -32.7416) (-32.162, -32.9341) (-32.162, -34.0886) knots -1 -1 -1 -1 0 0 0 0
  spline S88 degree 3 poles (-32.162, -34.0886) (-32.162, -35.2302) (-32.2005, -35.4483) (-32.5084, -36.0127) knots -1 -1 -1 -1 0 0 0 0
  spline S89 degree 3 poles (-17.7949, -12.0889) (-17.8462, -12.3326) (-17.9103, -12.5763) (-17.9488, -12.6405) knots -1 -1 -1 -1 0 0 0 0
  spline S90 degree 3 poles (-17.9488, -12.6405) (-17.9745, -12.6918) (-18.3978, -12.7303) (-18.8981, -12.7303) knots -1 -1 -1 -1 0 0 0 0
  line L18 (-18.8981, -12.7303) -> (-19.7832, -12.7303)
  line L19 (-19.7832, -12.7303) -> (-19.7832, -3.366)
  line L20 (-19.7832, -3.366) -> (-3.4919, -3.366)
  line L21 (-3.4919, -3.366) -> (-3.4919, -5.0079)
  spline S91 degree 3 poles (-3.4919, -5.0079) (-3.4919, -5.9059) (-3.5304, -6.9321) (-3.5688, -7.3041) knots -1 -1 -1 -1 0 0 0 0
  line L22 (-3.5688, -7.3041) -> (-3.6586, -7.9583)
  line L23 (-3.6586, -7.9583) -> (-4.3898, -7.458)
  spline S92 degree 3 poles (-4.3898, -7.458) (-8.2382, -4.8412) (-13.0358, -5.3928) (-16.0375, -8.805) knots -1 -1 -1 -1 0 0 0 0
  spline S93 degree 3 poles (-16.0375, -8.805) (-16.7302, -9.5874) (-17.6281, -11.2679) (-17.7949, -12.0889) knots -1 -1 -1 -1 0 0 0 0
  spline S94 degree 3 poles (-4.7105, -13.6026) (-4.4668, -15.7705) (-5.9805, -17.9768) (-8.1099, -18.5669) knots -1 -1 -1 -1 0 0 0 0
  spline S95 degree 3 poles (-8.1099, -18.5669) (-9.8288, -19.0415) (-11.6504, -18.5669) (-12.8947, -17.3226) knots -1 -1 -1 -1 0 0 0 0
  spline S96 degree 3 poles (-12.8947, -17.3226) (-15.178, -15.0393) (-14.4981, -11.0242) (-11.599, -9.7542) knots -1 -1 -1 -1 0 0 0 0
  spline S97 degree 3 poles (-11.599, -9.7542) (-9.8929, -8.9974) (-7.6609, -9.3437) (-6.2242, -10.6008) knots -1 -1 -1 -1 0 0 0 0
  spline S98 degree 3 poles (-6.2242, -10.6008) (-5.5187, -11.2166) (-4.826, -12.5892) (-4.7105, -13.6026) knots -1 -1 -1 -1 0 0 0 0
  spline S99 degree 3 poles (-18.6415, -37.6932) (-19.0648, -38.3217) (-19.8986, -38.9503) (-20.5657, -39.1299) knots -1 -1 -1 -1 0 0 0 0
  spline S100 degree 3 poles (-20.5657, -39.1299) (-20.8094, -39.2069) (-21.2071, -39.271) (-21.4508, -39.271) knots -1 -1 -1 -1 0 0 0 0
  spline S101 degree 3 poles (-21.4508, -39.271) (-21.9254, -39.2838) (-29.0449, -38.3987) (-29.1347, -38.3089) knots -1 -1 -1 -1 0 0 0 0
  spline S102 degree 3 poles (-29.1347, -38.3089) (-29.1603, -38.2833) (-29.032, -37.783) (-28.8396, -37.1929) knots -1 -1 -1 -1 0 0 0 0
  spline S103 degree 3 poles (-28.8396, -37.1929) (-28.4163, -35.8588) (-28.288, -34.2553) (-28.4933, -32.9212) knots -1 -1 -1 -1 0 0 0 0
  spline S104 degree 3 poles (-28.4933, -32.9212) (-28.5959, -32.344) (-28.6087, -31.895) (-28.5446, -31.8309) knots -1 -1 -1 -1 0 0 0 0
  spline S105 degree 3 poles (-28.5446, -31.8309) (-28.4804, -31.7667) (-26.8385, -31.6769) (-24.9015, -31.6384) knots -1 -1 -1 -1 0 0 0 0
  spline S106 degree 3 poles (-24.9015, -31.6384) (-21.4636, -31.5615) (-21.3738, -31.5615) (-20.6298, -31.8437) knots -1 -1 -1 -1 0 0 0 0
  spline S107 degree 3 poles (-20.6298, -31.8437) (-18.2439, -32.7545) (-17.2561, -35.6792) (-18.6415, -37.6932) knots -1 -1 -1 -1 0 0 0 0
  spline S108 degree 3 poles (-25.8123, -18.2719) (-25.8123, -18.6311) (-26.0175, -19.4905) (-26.2612, -20.1447) knots -1 -1 -1 -1 0 0 0 0
  spline S109 degree 3 poles (-26.2612, -20.1447) (-26.3382, -20.3628) (-26.351, -20.3628) (-27.7236, -19.7984) knots -1 -1 -1 -1 0 0 0 0
  spline S110 degree 3 poles (-27.7236, -19.7984) (-29.2758, -19.157) (-32.4314, -18.1821) (-33.5474, -17.9897) knots -1 -1 -1 -1 0 0 0 0
  spline S111 degree 3 poles (-33.5474, -17.9897) (-34.0221, -17.8999) (-34.4069, -17.7972) (-34.4069, -17.7459) knots -1 -1 -1 -1 0 0 0 0
  spline S112 degree 3 poles (-34.4069, -17.7459) (-34.4069, -17.4252) (-33.8553, -16.3349) (-33.4448, -15.8474) knots -1 -1 -1 -1 0 0 0 0
  spline S113 degree 3 poles (-33.4448, -15.8474) (-32.8162, -15.0906) (-32.0722, -14.7571) (-31.123, -14.8084) knots -1 -1 -1 -1 0 0 0 0
  line L24 (-31.123, -14.8084) -> (-30.4174, -14.8468)
  line L25 (-30.4174, -14.8468) -> (-30.1352, -14.1413)
  spline S114 degree 3 poles (-30.1352, -14.1413) (-29.8017, -13.3203) (-29.8274, -13.3203) (-28.1597, -13.8335) knots -1 -1 -1 -1 0 0 0 0
  spline S115 degree 3 poles (-28.1597, -13.8335) (-26.9539, -14.2055) (-26.9283, -14.2311) (-27.3516, -15.3086) knots -1 -1 -1 -1 0 0 0 0
  spline S116 degree 3 poles (-27.3516, -15.3086) (-27.5055, -15.6678) (-27.5953, -15.9885) (-27.5825, -16.0014) knots -1 -1 -1 -1 0 0 0 0
  spline S117 degree 3 poles (-27.5825, -16.0014) (-27.5568, -16.0142) (-27.3003, -16.1553) (-27.0052, -16.3092) knots -1 -1 -1 -1 0 0 0 0
  spline S118 degree 3 poles (-27.0052, -16.3092) (-26.3767, -16.6171) (-25.8123, -17.5663) (-25.8123, -18.2719) knots -1 -1 -1 -1 0 0 0 0
  line L26 (0, -45) -> (0, 0)
  line L27 (0, 0) -> (-45, 0)
  line L28 (-45, 0) -> (-45, -45)
  line L29 (-45, -45) -> (0, -45)
  circle A0 centre (-4, -22.5) radius 1.5
  circle A1 centre (-41, -21.9021) radius 1.5
  dimension "d7" = 3
  dimension "d8" = 3
  measures "d7" diameter of A0
  measures "d8" diameter of A1
extrude "Extrude3" cut sketch "Sketch3" against normal blind 10 contours A0 | A1